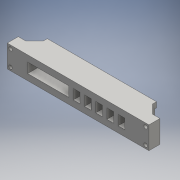
# Autodesk Inventor part: OttosDIY_Testing
Saved by Autodesk Inventor 2016 (Build 200138000, 138)
## iProperties
Created: 2018-04-06
Part Number: OttosDIY_Testing
Material: Generic
Document SubType Name: Modeling
Designer: suku
Density: 1 g/cm^3
Appearance: Default
Author: suku
Autodesk Inventor part; units mm, degrees
ref_plane "YZ Plane" through (0, 0, 0) normal (1, 0, 0) x (0, 1, 0)
ref_plane "XZ Plane" through (0, 0, 0) normal (0, 1, 0) x (-1, 0, 0)
ref_plane "XY Plane" through (0, 0, 0) normal (0, 0, 1) x (1, 0, 0)
sketch "Sketch1" plane through (0, 0, 0) normal (0, 1, 0) x (-1, 0, 0)
  line L0 (0, 0) -> (128.5, 0)
  line L1 (128.5, 0) -> (128.5, -20.32)
  line L2 (128.5, -20.32) -> (0, -20.32)
  line L3 (0, -20.32) -> (0, 0)
  dimension "d0" = 20.32
  dimension "d1" = 128.5
  constraints: 8 end point, 2 parallel, 1 horizontal, 1 perpendicular
  measures "d0" distance of L0.end L1.end
  measures "d1" distance of L1.end L2.end
extrude "Extrusion1" add sketch "Sketch1" along normal blind 10
sketch "Sketch2" plane through (0, 10, 0) normal (0, 1, 0) x (1, 0, 0)
  line L0 (-128.5, 0) -> (0, 0) projected
  line L1 (0, 0) -> (0, 20.32) projected
  line L2 (0, 20.32) -> (-128.5, 20.32) projected
  line L3 (-128.5, 20.32) -> (-128.5, 0) projected
  line L4 (-128.5, 0) -> (0, 0) projected
  line L5 (0, 20.32) -> (-128.5, 20.32) projected
  line L6 (-14.72, 0) -> (-113.78, 0)
  line L7 (-113.78, 0) -> (-113.78, 20.32)
  line L8 (-113.78, 20.32) -> (-14.72, 20.32)
  line L9 (-14.72, 20.32) -> (-14.72, 0)
  line L10 (-128.5, 20.32) -> (-113.78, 20.32)
  line L11 (-128.5, 20.32) -> (0, 20.32) projected
  line L12 (-14.72, 20.32) -> (0, 20.32)
  line L13 (-128.5, 10.16) -> (-113.78, 10.16)
  line L14 (-14.72, 10.16) -> (0, 10.16)
  dimension "d19" = 99.06
  constraints: 16 end point, 4 midpoint, 2 collinear, 2 horizontal, 2 parallel, 2 point on line, 1 perpendicular
  measures "d19" distance between parallel lines of L7 L9
extrude "Extrusion2" add sketch "Sketch2" along normal blind 10 contours L7 L2 L9 L0
sketch "Sketch3" plane through (0, 10, 0) normal (0, 1, 0) x (1, 0, 0)
  line L0 (-113.78, 0) -> (-113.78, 20.32) projected
  line L1 (-113.78, 20.32) -> (-128.5, 20.32) projected
  line L2 (-128.5, 20.32) -> (-128.5, 0) projected
  line L3 (-128.5, 0) -> (-113.78, 0) projected
  line L4 (-14.72, 20.32) -> (-14.72, 0) projected
  line L5 (-14.72, 0) -> (0, 0) projected
  line L6 (0, 0) -> (0, 20.32) projected
  line L7 (0, 20.32) -> (-14.72, 20.32) projected
  line L8 (-113.78, 20.32) -> (-128.5, 20.32) projected
  line L9 (-128.5, 0) -> (-125.5, 0)
  line L10 (-125.5, 0) -> (-125.5, 20.32)
  line L11 (-125.5, 20.32) -> (-128.5, 20.32)
  line L12 (-128.5, 20.32) -> (-128.5, 0)
  line L13 (-128.5, 20.32) -> (0, 20.32) projected
  line L14 (0, 0) -> (-3, 0)
  line L15 (-3, 0) -> (-3, 20.32)
  line L16 (-3, 20.32) -> (0, 20.32)
  line L17 (0, 20.32) -> (0, 0)
  line L18 (-125.5, 0) -> (-3, 0)
  line L19 (-3, 0) -> (-3, 3)
  line L20 (-3, 3) -> (-125.5, 3)
  line L21 (-125.5, 3) -> (-125.5, 0)
  line L22 (-125.5, 20.32) -> (-3, 20.32)
  line L23 (-3, 20.32) -> (-3, 17.32)
  line L24 (-3, 17.32) -> (-125.5, 17.32)
  line L25 (-125.5, 17.32) -> (-125.5, 20.32)
  dimension "d8" = 3
  dimension "d9" = 3
  dimension "d10" = 3
  dimension "d11" = 3
  constraints: 32 end point, 8 parallel, 4 horizontal, 4 perpendicular, 4 point on line
  measures "d8" distance of L11.end L10.end
  measures "d9" distance of L15.end L16.end
  measures "d10" distance of L19.end L18.end
  measures "d11" distance of L22.end L23.end
hole "Hole1" at (-125.5, 10, -3) at (-125.5, 10, -17.32) at (-3, 10, -17.32) at (-3, 10, -3) direction (0, -1, 0) diameter 3.2 end through all
sketch "Sketch4" plane through (0, 20, 0) normal (0, 1, 0) x (1, 0, 0)
  line L0 (-14.72, 20.32) -> (-14.72, 0) projected
  line L1 (-14.72, 10.16) -> (-113.78, 10.16)
  line L2 (-113.78, 20.32) -> (-113.78, 0) projected
  line L3 (-27.88, 5.66) -> (-21.88, 5.66)
  line L4 (-21.88, 5.66) -> (-21.88, 14.66)
  line L5 (-21.88, 14.66) -> (-27.88, 14.66)
  line L6 (-27.88, 14.66) -> (-27.88, 5.66)
  line L7 (-27.88, 5.66) -> (-21.88, 14.66) construction
  line L8 (-21.88, 5.66) -> (-27.88, 14.66) construction
  line L9 (-38.04, 5.66) -> (-32.04, 5.66)
  line L10 (-32.04, 5.66) -> (-32.04, 14.66)
  line L11 (-32.04, 14.66) -> (-38.04, 14.66)
  line L12 (-38.04, 14.66) -> (-38.04, 5.66)
  line L13 (-38.04, 5.66) -> (-32.04, 14.66) construction
  line L14 (-32.04, 5.66) -> (-38.04, 14.66) construction
  line L15 (-48.2, 5.66) -> (-42.2, 5.66)
  line L16 (-42.2, 5.66) -> (-42.2, 14.66)
  line L17 (-42.2, 14.66) -> (-48.2, 14.66)
  line L18 (-48.2, 14.66) -> (-48.2, 5.66)
  line L19 (-48.2, 5.66) -> (-42.2, 14.66) construction
  line L20 (-42.2, 5.66) -> (-48.2, 14.66) construction
  line L21 (-58.36, 5.66) -> (-52.36, 5.66)
  line L22 (-52.36, 5.66) -> (-52.36, 14.66)
  line L23 (-52.36, 14.66) -> (-58.36, 14.66)
  line L24 (-58.36, 14.66) -> (-58.36, 5.66)
  line L25 (-58.36, 5.66) -> (-52.36, 14.66) construction
  line L26 (-52.36, 5.66) -> (-58.36, 14.66) construction
  line L27 (-68.52, 5.66) -> (-62.52, 5.66)
  line L28 (-62.52, 5.66) -> (-62.52, 14.66)
  line L29 (-62.52, 14.66) -> (-68.52, 14.66)
  line L30 (-68.52, 14.66) -> (-68.52, 5.66)
  line L31 (-68.52, 5.66) -> (-62.52, 14.66) construction
  line L32 (-62.52, 5.66) -> (-68.52, 14.66) construction
  line L33 (-78.68, 5.66) -> (-72.68, 5.66)
  line L34 (-72.68, 5.66) -> (-72.68, 14.66)
  line L35 (-72.68, 14.66) -> (-78.68, 14.66)
  line L36 (-78.68, 14.66) -> (-78.68, 5.66)
  line L37 (-78.68, 5.66) -> (-72.68, 14.66) construction
  line L38 (-72.68, 5.66) -> (-78.68, 14.66) construction
  line L39 (-72.68, 14.66) -> (-109.97, 14.66)
  line L40 (-109.97, 14.66) -> (-109.97, 5.66)
  line L41 (-109.97, 5.66) -> (-72.68, 5.66)
  line L42 (-72.68, 5.66) -> (-72.68, 14.66)
  point P0 (-24.88, 10.16)
  point P1 (-35.04, 10.16)
  point P2 (-45.2, 10.16)
  point P3 (-55.36, 10.16)
  point P4 (-65.52, 10.16)
  point P5 (-75.68, 10.16)
  dimension "d22" = 6
  dimension "d23" = 9
  dimension "d24" = 10.16
  dimension "d25" = 6
  dimension "d26" = 9
  dimension "d27" = 10.16
  dimension "d28" = 6
  dimension "d29" = 9
  dimension "d30" = 6
  dimension "d31" = 9
  dimension "d32" = 6
  dimension "d33" = 9
  dimension "d34" = 6
  dimension "d35" = 9
  dimension "d36" = 10.16
  dimension "d37" = 10.16
  dimension "d38" = 10.16
  dimension "d39" = 10.16
  dimension "d41" = 3.81
  constraints: 82 end point, 14 midpoint, 14 parallel, 7 perpendicular, 6 point on line, 1 horizontal
  measures "d22" distance of L3.start L3.end
  measures "d23" distance of L4.end L3.end
  measures "d24" distance from line of point (-24.88, 10.16) L0
  measures "d25" distance of L9.start L9.end
  measures "d26" distance of L10.end L9.end
  measures "d27" distance of point (-35.04, 10.16) point (-24.88, 10.16)
  measures "d28" distance of L15.start L15.end
  measures "d29" distance of L16.end L15.end
  measures "d30" distance of L21.start L21.end
  measures "d31" distance of L22.end L21.end
  measures "d32" distance of L27.start L27.end
  measures "d33" distance of L28.end L27.end
  measures "d34" distance of L33.start L33.end
  measures "d35" distance of L34.end L33.end
  measures "d36" distance of point (-45.2, 10.16) point (-35.04, 10.16)
  measures "d37" distance of point (-45.2, 10.16) point (-55.36, 10.16)
  measures "d38" distance of point (-65.52, 10.16) point (-55.36, 10.16)
  measures "d39" distance of point (-75.68, 10.16) point (-65.52, 10.16)
  measures "d41" distance between parallel lines of L2 L40
extrude "Extrusion3" cut sketch "Sketch4" against normal through all
sketch "Sketch5" plane through (0, 20, 0) normal (0, 1, 0) x (1, 0, 0)
  line L0 (-14.72, 0) -> (-14.72, 20.32) projected
  line L1 (-113.78, 20.32) -> (-113.78, 0) projected
  line L2 (-14.72, 0) -> (-113.78, 20.32)
  line L3 (-113.78, 0) -> (-14.72, 20.32)
  line L4 (-111.875, 13.335) -> (-111.875, 6.985)
  line L5 (-111.875, 6.985) -> (-16.625, 6.985)
  line L6 (-16.625, 6.985) -> (-16.625, 13.335)
  line L7 (-16.625, 13.335) -> (-111.875, 13.335)
  line L8 (-111.875, 13.335) -> (-16.625, 6.985) construction
  line L9 (-111.875, 6.985) -> (-16.625, 13.335) construction
  point P0 (0, 0)
  point P1 (-64.25, 10.16)
  dimension "d44" = 95.25
  dimension "d45" = 6.35
  constraints: 16 end point, 3 midpoint, 2 parallel, 1 perpendicular, 1 vertical
  measures "d44" distance of L5.end L4.end
  measures "d45" distance of L5.end L6.end
hole "Hole2" at (-16.625, 20, -13.335) at (-16.625, 20, -6.985) at (-111.875, 20, -13.335) at (-111.875, 20, -6.985) direction (0, -1, 0) diameter 2.2 depth 16 tip angle 118
chamfer "Chamfer1" distance 8 angle 45 2 edges at (-14.72, 10, -10.16) (-113.78, 10, -10.16)
sketch "Sketch6" plane through (0, 20, 0) normal (0, 1, 0) x (1, 0, 0)
  line L0 (-14.72, 0) -> (-14.72, 20.32) projected
  line L1 (-113.78, 20.32) -> (-121.78, 20.32) projected
  line L2 (-14.72, 20.32) -> (-113.78, 20.32)
  line L3 (-113.78, 20.32) -> (-113.78, 15.49)
  line L4 (-113.78, 15.49) -> (-14.72, 15.49)
  line L5 (-14.72, 15.49) -> (-14.72, 20.32)
  line L6 (-113.78, 0) -> (-14.72, 0)
  line L7 (-14.72, 0) -> (-14.72, 4.83)
  line L8 (-14.72, 4.83) -> (-113.78, 4.83)
  line L9 (-113.78, 4.83) -> (-113.78, 0)
  point P0 (0, 0)
  dimension "d56" = 10.66
  constraints: 16 end point, 4 parallel, 3 perpendicular, 2 collinear
  measures "d56" distance between parallel lines of L8 L4
extrude "Extrusion4" add sketch "Sketch6" along normal blind 1.6
body "Solid1"
